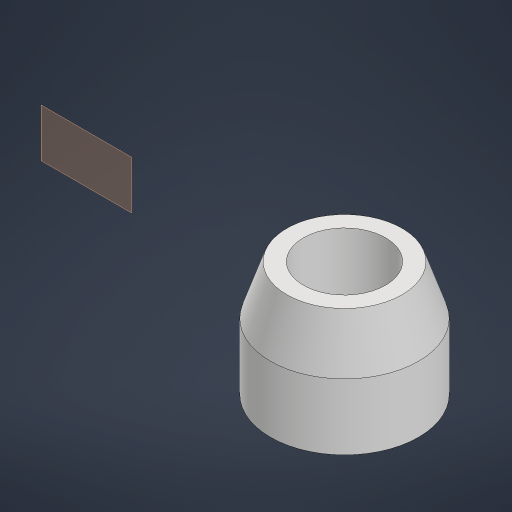
# Autodesk Inventor part: LimitedView_Parts
Saved by Autodesk Inventor 2024.2 (Build 282272000, 272)
## iProperties
Created: 2024-01-10
Part Number: LimitedView_Parts
Material: 一般
Document SubType Name: Modeling
Designer: Hanaoka
Density: 1 g/cm^3
Appearance: 既定
Author: Hanaoka
Autodesk Inventor part; units mm, degrees
ref_plane "YZ Plane" through (0, 0, 0) normal (1, 0, 0) x (0, 1, 0)
ref_plane "XZ Plane" through (0, 0, 0) normal (0, 1, 0) x (-1, 0, 0)
ref_plane "XY Plane" through (0, 0, 0) normal (0, 0, 1) x (1, 0, 0)
ref_plane "作業平面1" through (-45.0235, 27.1998, 9.5426) normal (0, 0, 1) x (1, 0, 0)
sketch "スケッチ2" plane through (0, 0, 0) normal (0, 0, 1) x (1, 0, 0)
  line L0 (7.5, 21) -> (7.5, 6)
  line L1 (7.5, 6) -> (11, 6)
  line L2 (11, 6) -> (11, 0)
  line L3 (11, 0) -> (13.5, 0)
  line L4 (13.5, 0) -> (13.5, 12)
  line L5 (-2.7, 0) -> (16.2, 0) projected
  line L6 (0, -4.2) -> (0, 25.2) projected
  line L7 (7.5, 21) -> (10.5, 21)
  line L8 (10.5, 21) -> (13.5, 12)
  point P0 (0, 0)
  point P1 (11, 3)
  dimension "d5" = 11
  dimension "d6" = 6
  dimension "d8" = 7.5
  dimension "d9" = 2.5
  dimension "d10" = 12
  dimension "d11" = 15
  dimension "d13" = 3
  constraints: 14 end point, 2 parallel, 2 vertical, 1 horizontal, 1 midpoint, 1 perpendicular, 1 point on line
  measures "d5" distance from line of point (0, 0) L2
  measures "d6" distance of L1.end L2.end
  measures "d8" distance from line of point (0, 0) L0
  measures "d9" distance of L2.end L3.end
  measures "d10" distance of L3.end L4.end
  measures "d11" distance of L0.start L0.end
  measures "d13" distance of L0.start L7.end
revolve "回転1" add sketch "スケッチ2" angle 360 about axis through (0, -10, 0) along (0, 1, 0)
